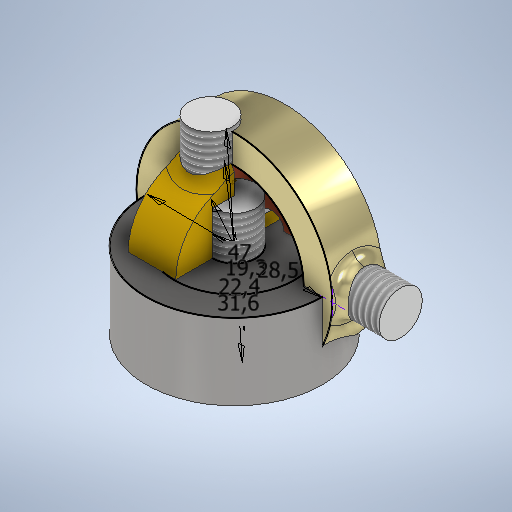
# Autodesk Inventor part: RBSDet
Saved by Autodesk Inventor 2025.2 (Build 292293000, 293)
## iProperties
Created: 2026-01-28
Part Number: RBSDet
Material: Generisch
Document SubType Name: Modeling
Designer: schum
Density: 1 g/cm^3
Appearance: Vorgabe
Author: schum
Autodesk Inventor part; units mm, degrees
ref_plane "YZ Plane" through (0, 0, 0) normal (1, 0, 0) x (0, 1, 0)
sketch "Skizze1" plane through (0, 0, 0) normal (0, 1, 0) x (-1, 0, 0)
  circle A0 centre (0, 0) radius 21.3
  circle A1 centre (0, 0) radius 12
  circle A2 centre (0, 0) radius 3.5
  dimension "d0" = 42.6
  dimension "d1" = 24
  dimension "d6" = 7
  constraints: 3 centre point, 3 coincident
  measures "d0" diameter of A0
  measures "d1" diameter of A1
  measures "d6" diameter of A2
extrude "Extrusion1" [suppressed]
extrude "Extrusion2" [suppressed]
extrude "Extrusion3" [suppressed]
thread "Gewinde1" size "M7x1" class "6g" standard "ANSI Metric M Profile" full length
sketch "Skizze2" plane through (0, 0, 0) normal (1, 0, 0) x (0, 1, 0)
  circle A0 centre (0, 0) radius 9.45
  circle A1 centre (0, 0) radius 5.85
  point P0 (0, 9.45)
  dimension "d11" = 18.9
  dimension "d12" = 11.7
  constraints: 2 coincident, 1 centre point, 1 vertical alignment, 2 other
  measures "d12" diameter of A1
extrude "Extrusion4" add sketch "Skizze2" against normal blind 7.7
extrude "Extrusion5" add sketch "Skizze2" against normal blind 7.3 contours A1
ref_plane "Arbeitsebene1" through (0, 0, 9.45) normal (0, 0, 1) x (1, 0, 0)
sketch "Skizze3" plane through (0, 0, 9.45) normal (0, 0, 1) x (1, 0, 0)
  circle A0 centre (-3.85, 0) radius 3.5
  point P0 (0, 0)
  dimension "d17" = 7
  constraints: 1 centre point
  measures "d17" diameter of A0
extrude "Extrusion6" add sketch "Skizze3" along normal blind 7
extrude "Extrusion7" add sketch "Skizze3" against normal blind 2
fillet "Flächenabrundung1" radius 2 2 edges at (-3.851, 3.5, 8.778) (-3.8522, -3.5, 8.778)
thread "Gewinde2" size "M7x1" class "6g" standard "ANSI Metric M Profile" full length
sketch "Skizze4" plane through (0, 0, 0) normal (0, 1, 0) x (-1, 0, 0)
  circle A0 centre (0, 0) radius 2
  circle A1 centre (0, 0) radius 15.8
  circle A2 centre (0, 0) radius 11.2
  point P0 (-15.8, 0)
  dimension "d26" = 31.6
  dimension "d25" = 4
  dimension "d27" = 22.4
  constraints: 3 coincident, 2 centre point, 1 horizontal alignment, 2 other
  measures "d25" diameter of A0
  measures "d27" diameter of A2
extrude "Extrusion8" add sketch "Skizze4" along normal blind 8.1 contours A1
extrude "Extrusion9" add sketch "Skizze4" along normal blind 6.7 contours A2
extrude "Extrusion10" cut sketch "Skizze4" along normal blind 6 contours A2
ref_plane "Arbeitsebene2" through (15.8, 0, 0) normal (1, 0, 0) x (0, 1, 0)
sketch "Skizze5" plane through (15.8, 0, 0) normal (1, 0, 0) x (0, 1, 0)
  circle A0 centre (4.05, 0) radius 3.5
  point P0 (0, 0)
  dimension "d34" = 7
  constraints: 1 centre point
  measures "d34" diameter of A0
extrude "Extrusion11" add sketch "Skizze5" along normal blind 7
extrude "Extrusion12" add sketch "Skizze5" against normal blind 2
fillet "Flächenabrundung2" radius 2 2 edges at (15.4075, 4.05, 3.5) (15.4075, 4.05, -3.5)
fillet "Flächenabrundung3" radius 1 1 edges at (11.2, 6.7, 0)
fillet "Flächenabrundung4" radius 2 1 edges at (11.2, 6, 0)
thread "Gewinde3" size "M7x1" class "6g" standard "ANSI Metric M Profile" full length
sketch "Skizze6" plane through (0, 0, 0) normal (0, 0, 1) x (1, 0, 0)
  circle A0 centre (0, 0) radius 14.25
  circle A1 centre (0, 0) radius 9.65
  circle A2 centre (0, 0) radius 3.5
  dimension "d44" = 28.5
  dimension "d45" = 19.3
  dimension "d46" = 7
  constraints: 3 centre point, 3 coincident
  measures "d44" diameter of A0
  measures "d45" diameter of A1
  measures "d46" diameter of A2
extrude "Extrusion13" add sketch "Skizze6" against normal blind 12.3 contours A0
extrude "Extrusion14" add sketch "Skizze6" against normal blind 12 contours A1
extrude "Extrusion15" add sketch "Skizze6" against normal blind 12 contours A2
extrude "Extrusion16" add sketch "Skizze6" along normal blind 7 contours A2
thread "Gewinde4" size "M7x1" class "6g" standard "ANSI Metric M Profile" full length
